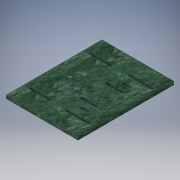
# Autodesk Inventor part: top frame 4x4
Saved by Autodesk Inventor 2017 (Build 210142000, 142)
## iProperties
Created: 2019-12-31
Part Number: top frame 4x4
Material: Nickel-Copper Alloy 400
Document SubType Name: Modeling
Designer: Admin
Density: 8.83 g/cm^3
Appearance: Green Polished
Mass: 208.506 g
Surface Area: 170.429 cm^2
Volume: 23.6134 cm^3
Author: Admin
Autodesk Inventor part; units mm, degrees
ref_plane "YZ Plane" through (0, 0, 0) normal (1, 0, 0) x (0, 1, 0)
ref_plane "XZ Plane" through (0, 0, 0) normal (0, 1, 0) x (-1, 0, 0)
ref_plane "XY Plane" through (0, 0, 0) normal (0, 0, 1) x (1, 0, 0)
sketch "Sketch1" plane through (0, 0, 0) normal (0, 1, 0) x (-1, 0, 0)
  line L0 (-38.1, -50.8) -> (38.1, -50.8)
  line L1 (38.1, -50.8) -> (38.1, 50.8)
  line L2 (38.1, 50.8) -> (-38.1, 50.8)
  line L3 (-38.1, 50.8) -> (-38.1, -50.8)
  line L4 (-38.1, -50.8) -> (38.1, 50.8) construction
  line L5 (38.1, -50.8) -> (-38.1, 50.8) construction
  point P0 (0, 0)
  dimension "d0" = 101.6
  dimension "d1" = 76.2
  constraints: 12 end point, 2 midpoint, 2 parallel, 1 horizontal, 1 perpendicular
  measures "d0" distance of L2.end L0.start
  measures "d1" distance of L0.start L0.end
extrude "Extrusion1" add sketch "Sketch1" along normal blind 3.175
sketch "Sketch2" plane through (0, 3.175, 0) normal (0, 1, 0) x (1, 0, 0)
  line L0 (-9.9878, -31.7793) -> (-30.8713, -31.7793) construction
  line L1 (-9.9878, -30.7915) -> (-30.8713, -30.7915)
  line L2 (-30.8713, -32.7672) -> (-9.9878, -32.7672)
  arc A0 (-9.9878, -32.7672) -> (-9.9878, -30.7915) centre (-9.9878, -31.7793) ccw
  arc A1 (-30.8713, -30.7915) -> (-30.8713, -32.7672) centre (-30.8713, -31.7793) ccw
  line L3 (7.9124, -32.7672) -> (32.6873, -32.7672) construction
  line L4 (7.9124, -33.755) -> (32.6873, -33.755)
  line L5 (32.6873, -31.7793) -> (7.9124, -31.7793)
  arc A2 (7.9124, -31.7793) -> (7.9124, -33.755) centre (7.9124, -32.7672) ccw
  arc A3 (32.6873, -33.755) -> (32.6873, -31.7793) centre (32.6873, -32.7672) ccw
  line L6 (20.2998, -22.4401) -> (12.582, -22.4401) construction
  line L7 (20.2998, -21.5321) -> (12.582, -21.5321)
  line L8 (12.582, -23.3481) -> (20.2998, -23.3481)
  arc A4 (20.2998, -23.3481) -> (20.2998, -21.5321) centre (20.2998, -22.4401) ccw
  arc A5 (12.582, -21.5321) -> (12.582, -23.3481) centre (12.582, -22.4401) ccw
  line L9 (20.2998, -13.3603) -> (4.4102, -13.3603) construction
  line L10 (20.2998, -12.2445) -> (4.4102, -12.2445)
  line L11 (4.4102, -14.4761) -> (20.2998, -14.4761)
  arc A6 (20.2998, -14.4761) -> (20.2998, -12.2445) centre (20.2998, -13.3603) ccw
  arc A7 (4.4102, -12.2445) -> (4.4102, -14.4761) centre (4.4102, -13.3603) ccw
  line L12 (-9.9878, 31.7793) -> (-30.8713, 31.7793) construction
  line L13 (-9.9878, 30.7915) -> (-30.8713, 30.7915)
  line L14 (-30.8713, 32.7672) -> (-9.9878, 32.7672)
  arc A8 (-9.9878, 30.7915) -> (-9.9878, 32.7672) centre (-9.9878, 31.7793) ccw
  arc A9 (-30.8713, 32.7672) -> (-30.8713, 30.7915) centre (-30.8713, 31.7793) ccw
  line L15 (7.9124, 32.7672) -> (32.6873, 32.7672) construction
  line L16 (7.9124, 33.755) -> (32.6873, 33.755)
  line L17 (32.6873, 31.7793) -> (7.9124, 31.7793)
  arc A10 (7.9124, 33.755) -> (7.9124, 31.7793) centre (7.9124, 32.7672) ccw
  arc A11 (32.6873, 31.7793) -> (32.6873, 33.755) centre (32.6873, 32.7672) ccw
  line L18 (20.2998, 22.4401) -> (12.582, 22.4401) construction
  line L19 (20.2998, 21.5321) -> (12.582, 21.5321)
  line L20 (12.582, 23.3481) -> (20.2998, 23.3481)
  arc A12 (20.2998, 21.5321) -> (20.2998, 23.3481) centre (20.2998, 22.4401) ccw
  arc A13 (12.582, 23.3481) -> (12.582, 21.5321) centre (12.582, 22.4401) ccw
  line L21 (20.2998, 13.3603) -> (4.4102, 13.3603) construction
  line L22 (20.2998, 12.2445) -> (4.4102, 12.2445)
  line L23 (4.4102, 14.4761) -> (20.2998, 14.4761)
  arc A14 (20.2998, 12.2445) -> (20.2998, 14.4761) centre (20.2998, 13.3603) ccw
  arc A15 (4.4102, 14.4761) -> (4.4102, 12.2445) centre (4.4102, 13.3603) ccw
  point P0 (-20.4296, -31.7793)
  point P1 (20.2998, -32.7672)
  point P2 (16.4409, -22.4401)
  point P3 (12.355, -13.3603)
  point P4 (0, -25.2547)
  point P5 (-20.4296, 31.7793)
  point P6 (20.2998, 32.7672)
  point P7 (16.4409, 22.4401)
  point P8 (12.355, 13.3603)
  constraints: 64 end point, 32 point on circle, 16 centre point, 16 tangent, 5 parallel, 4 midpoint, 4 point on line, 1 horizontal
extrude "Extrusion2" cut sketch "Sketch2" against normal blind 3.175
body "Solid1"
